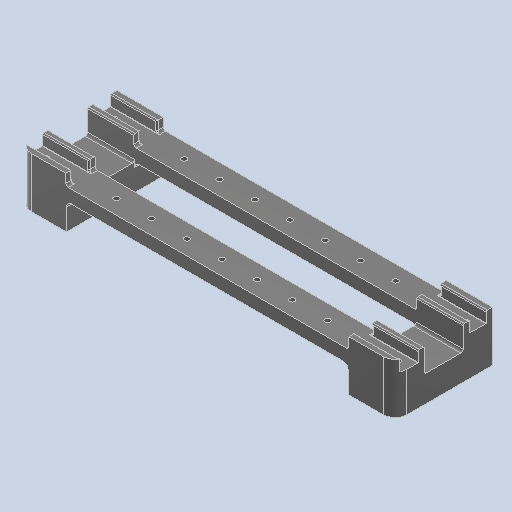
# Autodesk Inventor part: Part17
Saved by Autodesk Inventor 2024.3 (Build 283343010, 343A)
## iProperties
Created: 2025-06-26
Part Number: Part17
Material: 一般
Document SubType Name: Modeling
Designer: kshau
Density: 1 g/cm^3
Appearance: 滑らか - 黒
Author: kshau
Autodesk Inventor part; units mm, degrees
ref_plane "YZ Plane" through (0, 0, 0) normal (1, 0, 0) x (0, 1, 0)
ref_plane "XZ Plane" through (0, 0, 0) normal (0, 1, 0) x (-1, 0, 0)
ref_plane "XY Plane" through (0, 0, 0) normal (0, 0, 1) x (1, 0, 0)
sketch "スケッチ1" plane through (0, 0, 0) normal (0, 0, 1) x (1, 0, 0)
  line L0 (0, 0) -> (20, 0)
  line L1 (20, 0) -> (20, 21.49)
  line L2 (20, 21.49) -> (0, 21.49)
  line L3 (0, 21.49) -> (0, 0)
  line L4 (20, 16.79) -> (140, 16.79)
  line L5 (140, 16.79) -> (140, 11.29)
  line L6 (140, 11.29) -> (20, 11.29)
  line L7 (20, 11.29) -> (20, 16.79)
  line L8 (140, 21.49) -> (160, 21.49)
  line L9 (160, 21.49) -> (160, 0)
  line L10 (160, 0) -> (140, 0)
  line L11 (140, 0) -> (140, 21.49)
  line L12 (160, 0) -> (20, 0)
  point P0 (20, 11.29)
  dimension "d0" = 21.49
  dimension "d1" = 20
  dimension "d3" = 5.5
  dimension "d4" = 120
  dimension "d6" = 20
  dimension "d61" = 4.7
  dimension "d62" = 4.7
  constraints: 26 end point, 6 parallel, 3 horizontal, 3 perpendicular, 2 point on line, 1 collinear
  measures "d0" distance of L2.end L0.start
  measures "d1" distance between parallel lines of L3 L1
  measures "d3" distance between parallel lines of L6 L4
  measures "d4" distance of L4.start L4.end
  measures "d6" distance of L8.start L8.end
  measures "d61" distance between parallel lines of L2 L4
  measures "d62" distance between parallel lines of L4 L8
extrude "押し出し1" add sketch "スケッチ1" along normal blind 41.5 contours L3 L2 L1 L0 | L1 L4 L5 L6 | L11 L5 L8 L9 L10
sketch "スケッチ2" plane through (140, 21.49, 0) normal (0, 1, 0) x (1, 0, 0)
  line L0 (-140, 0) -> (-140, -41.5) projected
  line L1 (20, 0) -> (20, -41.5) projected
  line L2 (-140, -29) -> (20, -29)
  line L3 (20, -29) -> (20, -12.5)
  line L4 (20, -12.5) -> (-140, -12.5)
  line L5 (-140, -12.5) -> (-140, -29)
  line L6 (20, -41.5) -> (0, -41.5) projected
  line L7 (20, 0) -> (0, 0) projected
  dimension "d10" = 12.5
  dimension "d11" = 12.5
  constraints: 8 end point, 2 parallel, 2 point on line, 1 horizontal, 1 perpendicular
  measures "d10" distance between parallel lines of L6 L2
  measures "d11" distance between parallel lines of L7 L4
extrude "押し出し2" cut sketch "スケッチ2" against normal blind 10.2
sketch "スケッチ3" plane through (140, 21.49, 41.5) normal (0, 1, 0) x (1, 0, 0)
  line L0 (-140, 41.5) -> (-140, 0) projected
  line L1 (-140, 2.65) -> (20, 2.65)
  line L2 (20, 12.5) -> (20, 0) projected
  line L3 (20, 0) -> (0, 0) projected
  line L4 (20, 9.85) -> (-140, 9.85)
  line L5 (-140, 38.85) -> (20, 38.85)
  line L6 (20, 41.5) -> (20, 0) projected
  line L7 (20, 31.65) -> (-140, 31.65)
  line L8 (-120, 41.5) -> (-140, 41.5) projected
  line L9 (20, 41.5) -> (0, 41.5) projected
  line L10 (0.3, 0) -> (0.3, 41.5)
  line L11 (-120, 0) -> (-140, 0) projected
  line L12 (-120.3, 0) -> (-120.3, 41.5)
  line L13 (0, 0) -> (-120, 0) projected
  line L14 (-120, 41.5) -> (-120, 0) projected
  line L15 (-120, 0) -> (-120, 41.5)
  line L16 (0, 41.5) -> (-120, 41.5) projected
  line L17 (0, 41.5) -> (0, 0)
  point P0 (15, 26.15)
  point P1 (-120.3, 2.65)
  point P2 (-120.3, 9.85)
  point P3 (-120.3, 31.65)
  point P4 (-120.3, 38.85)
  point P5 (0.3, 38.85)
  point P6 (0.3, 31.65)
  point P7 (0.3, 9.85)
  point P8 (0.3, 2.65)
  point P9 (0, 38.85)
  point P10 (-120, 38.85)
  point P11 (-120, 2.65)
  point P12 (0, 2.65)
  point P13 (0, 9.85)
  point P14 (-120, 9.85)
  point P15 (-120, 31.65)
  point P16 (0, 31.65)
  dimension "d14" = 2.65
  dimension "d15" = 7.2
  dimension "d16" = 2.65
  dimension "d17" = 7.2
  dimension "d38" = 19.7
  dimension "d39" = 19.7
  constraints: 16 end point, 12 point on line, 5 perpendicular, 2 horizontal, 1 parallel
  measures "d14" distance between parallel lines of L3 L1
  measures "d15" distance between parallel lines of L1 L4
  measures "d16" distance between parallel lines of L8 L5
  measures "d17" distance between parallel lines of L5 L7
  measures "d38" distance between parallel lines of L6 L10
  measures "d39" distance between parallel lines of L0 L12
extrude "押し出し3" cut sketch "スケッチ3" against normal blind 4.7 contours L5 L12 L7 L0 | L8 L14 L5 L12 | L5 L14 L7 L12 | L4 L12 L1 L0 | L7 L14 L4 L12 | L5 L17 L7 L14 | L9 L10 L5 L17 | L4 L14 L1 L12 | L5 L10 L7 L17 | L1 L14 L11 L12 | L4 L17 L1 L14 | L7 L10 L4 L17 | L5 L6 L7 L10 | L4 L10 L1 L17 | L1 L10 L3 L17 | L4 L2 L1 L10
fillet "フィレット1" radius 5 2 edges at (160, 10.745, 41.5) (0, 10.745, 41.5)
sketch "スケッチ4" plane through (20, 16.79, 0) normal (0, 1, 0) x (1, 0, 0)
  line L0 (140, -2.65) -> (140, -9.85) projected
  line L1 (140, -6.25) -> (-20, -6.25)
  line L2 (-20, -9.85) -> (-20, -2.65) projected
  line L3 (-0.3, -38.85) -> (-19.4133, -38.85) projected
  line L4 (120.3, -31.65) -> (140, -31.65) projected
  line L5 (139.4, -35.25) -> (-20, -35.25)
  line L6 (-20, 0) -> (-20, -36.5) projected
  line L7 (-20, -31.65) -> (-0.3, -31.65) projected
  line L8 (140, -31.65) -> (140, -36.5) projected
  point P0 (135, -6.25)
  point P1 (139.4133, -38.85)
  point P2 (135, -35.25)
  point P3 (120, -35.25)
  point P4 (120, -6.25)
  point P5 (105, -35.25)
  point P6 (105, -6.25)
  point P7 (90, -35.25)
  point P8 (90, -6.25)
  point P9 (75, -35.25)
  point P10 (75, -6.25)
  point P11 (60, -35.25)
  point P12 (60, -6.25)
  point P13 (45, -35.25)
  point P14 (45, -6.25)
  point P15 (30, -35.25)
  point P16 (30, -6.25)
  point P17 (15, -35.25)
  point P18 (15, -6.25)
  point P19 (0, -35.25)
  point P20 (0, -6.25)
  point P21 (-15, -35.25)
  point P22 (-15, -6.25)
  dimension "d21" = 5
  dimension "d22" = 3.6
  dimension "d23" = 5
  dimension "d26" = 15
  constraints: 4 end point, 3 point on line, 2 horizontal, 2 midpoint, 21 other
  measures "d21" distance from line of L0 point (135, -6.25)
  measures "d22" distance between parallel lines of L7 L5
  measures "d26" distance of point (135, -35.25) point (120, -35.25)
hole "穴1" at (155, 16.79, 35.25) at (125, 16.79, 35.25) at (110, 16.79, 35.25) at (95, 16.79, 35.25) at (80, 16.79, 35.25) at (65, 16.79, 35.25) at (50, 16.79, 35.25) at (35, 16.79, 35.25) at (5, 16.79, 35.25) at (35, 16.79, 6.25) at (5, 16.79, 6.25) at (50, 16.79, 6.25) at (65, 16.79, 6.25) at (80, 16.79, 6.25) at (95, 16.79, 6.25) at (110, 16.79, 6.25) at (125, 16.79, 6.25) at (155, 16.79, 6.25) direction (0, -1, 0) diameter 2.3 end through all
sketch "スケッチ5" plane through (20, 11.29, 41.5) normal (0, -1, 0) x (1, 0, 0)
  circle A0 centre (15, -6.25) radius 1.15 projected
  circle A1 centre (15, -6.25) radius 3.2332
  line L0 (15, -6.25) -> (15, -3.0168)
  line L1 (13.3834, -3.45) -> (16.6166, -3.45)
  line L2 (16.6166, -3.45) -> (15, -6.25)
  line L3 (11.7668, -6.25) -> (13.3834, -3.45)
  line L4 (13.3834, -9.05) -> (11.7668, -6.25)
  line L5 (16.6166, -9.05) -> (13.3834, -9.05)
  line L6 (18.2332, -6.25) -> (16.6166, -9.05)
  line L7 (16.6166, -3.45) -> (18.2332, -6.25)
  circle A2 centre (15, -35.25) radius 1.15 projected
  circle A3 centre (15, -35.25) radius 3.2332
  line L8 (15, -35.25) -> (15, -32.0168)
  line L9 (16.6166, -32.45) -> (15, -35.25)
  line L10 (16.6166, -32.45) -> (13.3834, -32.45)
  line L11 (13.3834, -32.45) -> (11.7668, -35.25)
  line L12 (11.7668, -35.25) -> (13.3834, -38.05)
  line L13 (13.3834, -38.05) -> (16.6166, -38.05)
  line L14 (16.6166, -38.05) -> (18.2332, -35.25)
  line L15 (18.2332, -35.25) -> (16.6166, -32.45)
  line L16 (0, -41.5) -> (0, -12.5) projected
  line L17 (0, -41.5) -> (120, -41.5) projected
  line L18 (0, -41.5) -> (120, -41.5)
  line L19 (26.7668, -35.25) -> (28.3834, -38.05)
  line L20 (28.3834, -32.45) -> (26.7668, -35.25)
  line L21 (31.6166, -32.45) -> (28.3834, -32.45)
  line L22 (33.2332, -35.25) -> (31.6166, -32.45)
  line L23 (31.6166, -38.05) -> (33.2332, -35.25)
  line L24 (28.3834, -38.05) -> (31.6166, -38.05)
  line L25 (28.3834, -3.45) -> (31.6166, -3.45)
  line L26 (26.7668, -6.25) -> (28.3834, -3.45)
  line L27 (28.3834, -9.05) -> (26.7668, -6.25)
  line L28 (31.6166, -9.05) -> (28.3834, -9.05)
  line L29 (33.2332, -6.25) -> (31.6166, -9.05)
  line L30 (31.6166, -3.45) -> (33.2332, -6.25)
  line L31 (41.7668, -35.25) -> (43.3834, -38.05)
  line L32 (43.3834, -32.45) -> (41.7668, -35.25)
  line L33 (46.6166, -32.45) -> (43.3834, -32.45)
  line L34 (48.2332, -35.25) -> (46.6166, -32.45)
  line L35 (46.6166, -38.05) -> (48.2332, -35.25)
  line L36 (43.3834, -38.05) -> (46.6166, -38.05)
  line L37 (43.3834, -3.45) -> (46.6166, -3.45)
  line L38 (41.7668, -6.25) -> (43.3834, -3.45)
  line L39 (43.3834, -9.05) -> (41.7668, -6.25)
  line L40 (46.6166, -9.05) -> (43.3834, -9.05)
  line L41 (48.2332, -6.25) -> (46.6166, -9.05)
  line L42 (46.6166, -3.45) -> (48.2332, -6.25)
  line L43 (56.7668, -35.25) -> (58.3834, -38.05)
  line L44 (58.3834, -32.45) -> (56.7668, -35.25)
  line L45 (61.6166, -32.45) -> (58.3834, -32.45)
  line L46 (63.2332, -35.25) -> (61.6166, -32.45)
  line L47 (61.6166, -38.05) -> (63.2332, -35.25)
  line L48 (58.3834, -38.05) -> (61.6166, -38.05)
  line L49 (58.3834, -3.45) -> (61.6166, -3.45)
  line L50 (56.7668, -6.25) -> (58.3834, -3.45)
  line L51 (58.3834, -9.05) -> (56.7668, -6.25)
  line L52 (61.6166, -9.05) -> (58.3834, -9.05)
  line L53 (63.2332, -6.25) -> (61.6166, -9.05)
  line L54 (61.6166, -3.45) -> (63.2332, -6.25)
  line L55 (71.7668, -35.25) -> (73.3834, -38.05)
  line L56 (73.3834, -32.45) -> (71.7668, -35.25)
  line L57 (76.6166, -32.45) -> (73.3834, -32.45)
  line L58 (78.2332, -35.25) -> (76.6166, -32.45)
  line L59 (76.6166, -38.05) -> (78.2332, -35.25)
  line L60 (73.3834, -38.05) -> (76.6166, -38.05)
  line L61 (73.3834, -3.45) -> (76.6166, -3.45)
  line L62 (71.7668, -6.25) -> (73.3834, -3.45)
  line L63 (73.3834, -9.05) -> (71.7668, -6.25)
  line L64 (76.6166, -9.05) -> (73.3834, -9.05)
  line L65 (78.2332, -6.25) -> (76.6166, -9.05)
  line L66 (76.6166, -3.45) -> (78.2332, -6.25)
  line L67 (86.7668, -35.25) -> (88.3834, -38.05)
  line L68 (88.3834, -32.45) -> (86.7668, -35.25)
  line L69 (91.6166, -32.45) -> (88.3834, -32.45)
  line L70 (93.2332, -35.25) -> (91.6166, -32.45)
  line L71 (91.6166, -38.05) -> (93.2332, -35.25)
  line L72 (88.3834, -38.05) -> (91.6166, -38.05)
  line L73 (88.3834, -3.45) -> (91.6166, -3.45)
  line L74 (86.7668, -6.25) -> (88.3834, -3.45)
  line L75 (88.3834, -9.05) -> (86.7668, -6.25)
  line L76 (91.6166, -9.05) -> (88.3834, -9.05)
  line L77 (93.2332, -6.25) -> (91.6166, -9.05)
  line L78 (91.6166, -3.45) -> (93.2332, -6.25)
  line L79 (101.7668, -35.25) -> (103.3834, -38.05)
  line L80 (103.3834, -32.45) -> (101.7668, -35.25)
  line L81 (106.6166, -32.45) -> (103.3834, -32.45)
  line L82 (108.2332, -35.25) -> (106.6166, -32.45)
  line L83 (106.6166, -38.05) -> (108.2332, -35.25)
  line L84 (103.3834, -38.05) -> (106.6166, -38.05)
  line L85 (103.3834, -3.45) -> (106.6166, -3.45)
  line L86 (101.7668, -6.25) -> (103.3834, -3.45)
  line L87 (103.3834, -9.05) -> (101.7668, -6.25)
  line L88 (106.6166, -9.05) -> (103.3834, -9.05)
  line L89 (108.2332, -6.25) -> (106.6166, -9.05)
  line L90 (106.6166, -3.45) -> (108.2332, -6.25)
  point P0 (-20, -41.5)
  point P1 (0, -29)
  point P2 (103.3834, -3.45)
  point P3 (101.7668, -6.25)
  point P4 (106.6166, -9.05)
  point P5 (108.2332, -6.25)
  point P6 (88.3834, -3.45)
  point P7 (86.7668, -6.25)
  point P8 (91.6166, -9.05)
  point P9 (93.2332, -6.25)
  point P10 (101.7668, -35.25)
  point P11 (86.7668, -35.25)
  point P12 (71.7668, -35.25)
  point P13 (73.3834, -3.45)
  point P14 (71.7668, -6.25)
  point P15 (78.2332, -6.25)
  point P16 (58.3834, -3.45)
  point P17 (56.7668, -6.25)
  point P18 (61.6166, -9.05)
  point P19 (63.2332, -6.25)
  point P20 (43.3834, -3.45)
  point P21 (41.7668, -6.25)
  point P22 (46.6166, -9.05)
  point P23 (48.2332, -6.25)
  point P24 (56.7668, -35.25)
  point P25 (58.3834, -38.05)
  point P26 (61.6166, -38.05)
  point P27 (41.7668, -35.25)
  point P28 (43.3834, -38.05)
  point P29 (46.6166, -38.05)
  point P30 (26.7668, -35.25)
  point P31 (28.3834, -38.05)
  point P32 (31.6166, -38.05)
  point P33 (33.2332, -35.25)
  point P34 (31.6166, -32.45)
  point P35 (16.6166, -32.45)
  point P36 (11.7668, -35.25)
  point P37 (13.3834, -38.05)
  point P38 (16.6166, -38.05)
  point P39 (18.2332, -35.25)
  point P40 (28.3834, -3.45)
  point P41 (26.7668, -6.25)
  point P42 (28.3834, -9.05)
  point P43 (31.6166, -9.05)
  point P44 (33.2332, -6.25)
  point P45 (31.6166, -3.45)
  point P46 (13.3834, -3.45)
  point P47 (11.7668, -6.25)
  point P48 (13.3834, -9.05)
  point P49 (18.2332, -6.25)
  point P50 (16.6166, -3.45)
  dimension "d40" = 2.8
  dimension "d41" = 30
  dimension "d44" = 360
  dimension "d46" = 30
  dimension "d47" = 2.8
  dimension "d50" = 360
  dimension "d54" = 15
  constraints: 178 end point, 6 point on circle, 2 centre point, 2 coincident, 2 collinear, 2 perpendicular, 2 vertical, 1 horizontal, 253 other
  measures "d40" distance from line of A1.centre L1
  measures "d41" angle of L0 L2
  measures "d46" angle of L8 L9
  measures "d47" distance from line of L8.start L10
  measures "d54" distance of L12.start L19.start
extrude "押し出し4" cut sketch "スケッチ5" against normal blind 2 contours A0 L2 L7 L6 L5 L4 L3 L1 L0 | A0 L0 L1 L2 | A2 L9 L15 L14 L13 L12 L11 L10 L8 | A2 L8 L10 L9 | L20 L21 L22 L23 L24 L19 | L25 L30 L29 L28 L27 L26 | L32 L33 L34 L35 L36 L31 | L37 L42 L41 L40 L39 L38 | L44 L45 L46 L47 L48 L43 | L49 L54 L53 L52 L51 L50 | L56 L57 L58 L59 L60 L55 | L61 L66 L65 L64 L63 L62 | L68 L69 L70 L71 L72 L67 | L73 L78 L77 L76 L75 L74 | L80 L81 L82 L83 L84 L79 | L85 L90 L89 L88 L87 L86
fillet "フィレット2" radius 0.1 8 edges at (9.85, 16.79, 31.65) (10.1433, 16.79, 38.85) (9.85, 16.79, 2.65) (9.85, 16.79, 9.85) (150.15, 16.79, 2.65) (150.15, 16.79, 9.85) (150.15, 16.79, 31.65) (149.8567, 16.79, 38.85)
fillet "フィレット3" radius 1 20 edges at (150, 11.29, 12.5) (150, 11.29, 29) (140.3, 16.79, 38.8) (140.3, 16.79, 40.175) (140.3, 16.79, 31.7) (140.3, 16.79, 30.325) (140.3, 16.79, 1.325) (140.3, 16.79, 11.175) (140.3, 16.79, 2.7) (140.3, 16.79, 9.8) (10, 11.29, 12.5) (10, 11.29, 29) (19.7, 16.79, 40.175) (19.7, 16.79, 38.8) (19.7, 16.79, 30.325) (19.7, 16.79, 31.7) (19.7, 16.79, 2.7) (19.7, 16.79, 9.8) (19.7, 16.79, 1.325) (19.7, 16.79, 11.175)
fillet "フィレット4" radius 0.5 28 edges at (9.85, 21.49, 2.65) (9.85, 21.49, 9.85) (9.85, 21.49, 31.65) (10.1433, 21.49, 38.85) (150.15, 21.49, 2.65) (150.15, 21.49, 9.85) (150.15, 21.49, 29) (149.8567, 21.49, 38.85) (139.5236, 16.8153, 2.65) (20.4764, 16.8153, 2.65) (140.3, 19.64, 2.65) (139.5236, 16.8153, 9.85) (140.3, 19.64, 9.85) (150.15, 21.49, 31.65) (150.15, 21.49, 12.5) (139.5236, 16.8153, 38.85) (20.4764, 16.8153, 38.85) (140.3, 19.64, 38.85) (20.4764, 16.8153, 31.65) (139.5236, 16.8153, 31.65) (140.3, 19.64, 31.65) (9.85, 21.49, 12.5) (9.85, 21.49, 29) (19.7, 19.64, 2.65) (20.4764, 16.8153, 9.85) (19.7, 19.64, 9.85) (19.7, 19.64, 31.65) (19.7, 19.64, 38.85)
fillet "フィレット5" radius 2 4 edges at (20, 11.29, 35.25) (20, 11.29, 6.25) (140, 11.29, 35.25) (140, 11.29, 6.25)
